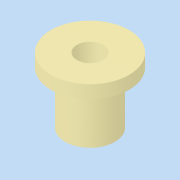
# Autodesk Inventor part: shoulderWasher
Saved by Autodesk Inventor 2017 (Build 210142000, 142)
## iProperties
Created: 2017-03-02
Part Number: shoulderWasher
Material: Nylon 6/6
Document SubType Name: Modeling
Designer: techn
Density: 1.13 g/cm^3
Appearance: Nylon 6
Author: techn
Autodesk Inventor part; units mm, degrees
ref_plane "YZ Plane" through (0, 0, 0) normal (1, 0, 0) x (0, 1, 0)
ref_plane "XZ Plane" through (0, 0, 0) normal (0, 1, 0) x (-1, 0, 0)
ref_plane "XY Plane" through (0, 0, 0) normal (0, 0, 1) x (1, 0, 0)
sketch "Sketch1" plane through (0, 0, 0) normal (0, 0, 1) x (1, 0, 0)
  line L0 (0, 0) -> (1.5113, 0)
  line L1 (1.5113, 0) -> (1.5113, 3.175)
  line L2 (1.5113, 3.175) -> (0, 3.175)
  line L3 (0, 3.175) -> (0, 0)
  line L4 (0, 3.175) -> (2.3749, 3.175)
  line L5 (2.3749, 3.175) -> (2.3749, 3.9624)
  line L6 (2.3749, 3.9624) -> (0, 3.9624)
  line L7 (0, 3.9624) -> (0, 3.175)
  dimension "d0" = 1.5113
  dimension "d1" = 2.3749
  dimension "d2" = 0.7874
  dimension "d3" = 3.175
  constraints: 16 end point, 4 parallel, 2 horizontal, 2 perpendicular
  measures "d0" distance between parallel lines of L3 L1
  measures "d1" distance between parallel lines of L7 L5
  measures "d2" distance between parallel lines of L6 L4
  measures "d3" distance between parallel lines of L2 L0
revolve "Revolution1" add sketch "Sketch1" angle 360 about axis through (0, 3.175, 0) along (0, -1, 0)
sketch "Sketch2" plane through (0, 3.9624, 0) normal (0, 1, 0) x (1, 0, 0)
  circle A0 centre (0, 0) radius 0.8001
  dimension "d5" = 1.6002
  constraints: 1 centre point, 1 coincident
  measures "d5" diameter of A0
extrude "Extrusion1" cut sketch "Sketch2" against normal blind 25.4
body "Solid1"
